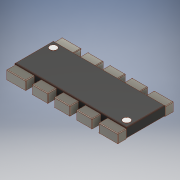
# Autodesk Inventor part: ResistorArray-3264
Saved by Autodesk Inventor 2018 (Build 220112000, 112)
## iProperties
Created: 2018-09-29
Part Number: ResistorArray-3264
Material: Copper
Document SubType Name: Modeling
Designer: Bradley
Density: 8.94 g/cm^3
Appearance: Copper - Satin
Author: Bradley
Autodesk Inventor part; units mm, degrees
ref_plane "YZ Plane" through (0, 0, 0) normal (1, 0, 0) x (0, 1, 0)
ref_plane "XZ Plane" through (0, 0, 0) normal (0, 1, 0) x (-1, 0, 0)
ref_plane "XY Plane" through (0, 0, 0) normal (0, 0, 1) x (1, 0, 0)
sketch "Sketch1" plane through (0, 0, 0) normal (0, 0, 1) x (1, 0, 0)
  line L0 (-3.2, -1.1) -> (3.2, -1.1)
  line L1 (3.2, -1.1) -> (3.2, 1.1)
  line L2 (3.2, 1.1) -> (-3.2, 1.1)
  line L3 (-3.2, 1.1) -> (-3.2, -1.1)
  line L4 (-3.2, -1.1) -> (3.2, 1.1) construction
  line L5 (3.2, -1.1) -> (-3.2, 1.1) construction
  point P0 (0, 0)
  dimension "d0" = 6.4
  dimension "d1" = 2.2
  constraints: 12 end point, 2 midpoint, 2 parallel, 1 horizontal, 1 perpendicular
  measures "d0" distance of L2.end L1.end
  measures "d1" distance of L2.end L0.start
extrude "Extrusion1" add sketch "Sketch1" along normal mid plane 0.55
sketch "Sketch2" plane through (0, 0, 0) normal (0, 0, 1) x (1, 0, 0)
  line L0 (-3.2, -1.1) -> (3.2, -1.1) projected
  line L1 (3.2, -1.1) -> (3.2, 1.1) projected
  line L2 (3.2, 1.1) -> (-3.2, 1.1) projected
  line L3 (-3.2, 1.1) -> (-3.2, -1.1) projected
  line L4 (3.2, 1.1) -> (-3.2, 1.1) projected
  line L5 (-3.19, 1.1) -> (-2.09, 1.1)
  line L6 (-2.09, 1.1) -> (-2.09, 1.6)
  line L7 (-2.09, 1.6) -> (-3.19, 1.6)
  line L8 (-3.19, 1.6) -> (-3.19, 1.1)
  line L9 (-3.19, -1.1) -> (-2.09, -1.1)
  line L10 (-2.09, -1.1) -> (-2.09, -1.6)
  line L11 (-2.09, -1.6) -> (-3.19, -1.6)
  line L12 (-3.19, -1.6) -> (-3.19, -1.1)
  line L13 (3.19, -1.1) -> (2.09, -1.1)
  line L14 (2.09, -1.1) -> (2.09, -1.6)
  line L15 (2.09, -1.6) -> (3.19, -1.6)
  line L16 (3.19, -1.6) -> (3.19, -1.1)
  line L17 (3.19, 1.1) -> (2.09, 1.1)
  line L18 (2.09, 1.1) -> (2.09, 1.6)
  line L19 (2.09, 1.6) -> (3.19, 1.6)
  line L20 (3.19, 1.6) -> (3.19, 1.1)
  line L21 (-1.72, 1.1) -> (-0.82, 1.1)
  line L22 (-0.82, 1.1) -> (-0.82, 1.6)
  line L23 (-0.82, 1.6) -> (-1.72, 1.6)
  line L24 (-1.72, 1.6) -> (-1.72, 1.1)
  line L25 (-3.2, -1.1) -> (3.2, -1.1) projected
  line L26 (-1.72, -1.1) -> (-0.82, -1.1)
  line L27 (-0.82, -1.1) -> (-0.82, -1.6)
  line L28 (-0.82, -1.6) -> (-1.72, -1.6)
  line L29 (-1.72, -1.6) -> (-1.72, -1.1)
  line L30 (-0.45, -1.1) -> (0.45, -1.1)
  line L31 (0.45, -1.1) -> (0.45, -1.6)
  line L32 (0.45, -1.6) -> (-0.45, -1.6)
  line L33 (-0.45, -1.6) -> (-0.45, -1.1)
  line L34 (0.45, 1.6) -> (-0.45, 1.6)
  line L35 (-0.45, 1.6) -> (-0.45, 1.1)
  line L36 (0.45, 1.1) -> (0.45, 1.6)
  line L37 (-0.45, 1.1) -> (0.45, 1.1)
  line L38 (0.82, -1.1) -> (1.72, -1.1)
  line L39 (1.72, -1.1) -> (1.72, -1.6)
  line L40 (1.72, -1.6) -> (0.82, -1.6)
  line L41 (0.82, -1.6) -> (0.82, -1.1)
  line L42 (1.72, 1.6) -> (0.82, 1.6)
  line L43 (0.82, 1.6) -> (0.82, 1.1)
  line L44 (1.72, 1.1) -> (1.72, 1.6)
  line L45 (0.82, 1.1) -> (1.72, 1.1)
  point P0 (0, 0)
  point P1 (0, 1.1)
  dimension "d4" = 1.1
  dimension "d5" = 0.9
  dimension "d6" = 3.2
  dimension "d9" = 1.27
  dimension "d18" = 0.01
  dimension "d19" = 0.01
  constraints: 80 end point, 14 point on line, 12 parallel, 7 horizontal, 6 perpendicular, 5 collinear, 4 equal length, 2 midpoint, 31 other
  measures "d4" distance of L6.end L7.end
  measures "d5" distance of L22.end L23.end
  measures "d6" distance between parallel lines of L11 L7
  measures "d9" distance of L26.end L30.end
  measures "d18" distance between parallel lines of L1 L20
  measures "d19" distance between parallel lines of L3 L8
extrude "Extrusion2" add sketch "Sketch2" along normal blind 0.2 and the other way blind 0.325 contours L0 L10 L11 L12 | L8 L7 L6 L2 | L0 L27 L28 L29 | L24 L23 L22 L2 | L0 L31 L32 L33 | L35 L34 L36 L2 | L0 L39 L40 L41 | L43 L42 L44 L2 | L0 L16 L15 L14 | L18 L19 L20 L2
sketch "Sketch3" plane through (0, 0, 0.275) normal (0, 0, 1) x (1, 0, 0)
  circle A0 centre (-2.85, 0.75) radius 0.2
  circle A1 centre (2.85, -0.75) radius 0.2
  line L0 (-3.2, -1.1) -> (3.2, -1.1) projected
  line L1 (3.2, -1.1) -> (3.2, 1.1) projected
  line L2 (3.2, 1.1) -> (-3.2, 1.1) projected
  line L3 (-3.2, 1.1) -> (-3.2, -1.1) projected
  circle A2 centre (-2.85, 0.75) radius 0.35 construction
  circle A3 centre (2.85, -0.75) radius 0.35 construction
  point P0 (0, 0)
  dimension "d20" = 0.4
  dimension "d21" = 0.7
  constraints: 4 centre point, 4 tangent, 2 coincident, 2 equal radius
  measures "d20" diameter of A0
  measures "d21" diameter of A2
extrude "Extrusion3" add sketch "Sketch3" along normal blind 0.01 contours A0 | A1
fillet "Fillet1" radius 0.03 110 edges at (-2.09, -1.35, -0.325) (-2.64, -1.6, -0.325) (-3.19, -1.35, -0.325) (-2.64, -1.1, -0.325) (-2.09, -1.6, -0.0625) (-2.64, -1.6, 0.2) (-3.19, -1.6, -0.0625) (-3.19, -1.35, 0.2) (-3.19, -1.1, -0.3) (-2.09, -1.1, -0.3) (-2.09, -1.35, 0.2) (-2.64, 1.1, -0.325) (-3.19, 1.35, -0.325) (-2.64, 1.6, -0.325) (-2.09, 1.35, -0.325) (-3.19, 1.35, 0.2) (-3.19, 1.6, -0.0625) (-3.19, 1.1, -0.3) (-2.64, 1.6, 0.2) (-2.09, 1.6, -0.0625) (-2.09, 1.35, 0.2) (-2.09, 1.1, -0.3) (1.27, -1.1, -0.325) (1.72, -1.35, -0.325) (1.27, -1.6, -0.325) (0.82, -1.35, -0.325) (1.72, -1.35, 0.2) (1.72, -1.6, -0.0625) (1.72, -1.1, -0.3) (1.27, -1.6, 0.2) (0.82, -1.6, -0.0625) (0.82, -1.35, 0.2) (0.82, -1.1, -0.3) (-1.27, 1.1, -0.325) (-1.72, 1.35, -0.325) (-1.27, 1.6, -0.325) (-0.82, 1.35, -0.325) (-1.72, 1.35, 0.2) (-1.72, 1.6, -0.0625) (-1.72, 1.1, -0.3) (-1.27, 1.6, 0.2) (-0.82, 1.6, -0.0625) (-0.82, 1.35, 0.2) (-0.82, 1.1, -0.3) (-0.82, -1.1, -0.3) (-1.27, -1.1, -0.325) (-1.72, -1.1, -0.3) (-1.72, -1.35, -0.325) (-0.82, -1.35, -0.325) (-1.27, -1.6, -0.325) (-0.82, -1.35, 0.2) (-0.82, -1.6, -0.0625) (-1.27, -1.6, 0.2) (-1.72, -1.6, -0.0625) (-1.72, -1.35, 0.2) (0, 1.1, -0.325) (-0.45, 1.35, -0.325) (0, 1.6, -0.325) (0.45, 1.35, -0.325) (-0.45, 1.1, -0.3) (-0.45, 1.35, 0.2) (-0.45, 1.6, -0.0625) (0, 1.6, 0.2) (0.45, 1.6, -0.0625) (0.45, 1.35, 0.2) (0.45, 1.1, -0.3) (0, -1.1, -0.325) (0.45, -1.35, -0.325) (0, -1.6, -0.325) (-0.45, -1.35, -0.325) (0.45, -1.35, 0.2) (0.45, -1.6, -0.0625) (0.45, -1.1, -0.3) (0, -1.6, 0.2) (-0.45, -1.6, -0.0625) (-0.45, -1.35, 0.2) (-0.45, -1.1, -0.3) (1.27, 1.1, -0.325) (0.82, 1.35, -0.325) (1.27, 1.6, -0.325) (1.72, 1.35, -0.325) (0.82, 1.35, 0.2) (0.82, 1.6, -0.0625) (0.82, 1.1, -0.3) (1.27, 1.6, 0.2) (1.72, 1.6, -0.0625) (1.72, 1.35, 0.2) (1.72, 1.1, -0.3) (2.09, 1.1, -0.3) (2.64, 1.1, -0.325) (3.19, 1.1, -0.3) (3.19, 1.35, -0.325) (2.09, 1.35, -0.325) (2.64, 1.6, -0.325) (2.09, 1.35, 0.2) (2.09, 1.6, -0.0625) (2.64, 1.6, 0.2) (3.19, 1.6, -0.0625) (3.19, 1.35, 0.2) (3.19, -1.1, -0.3) (2.64, -1.1, -0.325) (2.09, -1.1, -0.3) (2.09, -1.35, -0.325) (3.19, -1.35, -0.325) (2.64, -1.6, -0.325) (3.19, -1.35, 0.2) (3.19, -1.6, -0.0625) (2.64, -1.6, 0.2) (2.09, -1.6, -0.0625) (2.09, -1.35, 0.2)
fillet "Fillet2" radius 0.03 18 edges at (3.195, -1.1, -0.275) (1.905, -1.1, -0.275) (0.635, -1.1, -0.275) (-0.635, -1.1, -0.275) (-1.905, -1.1, -0.275) (-3.195, -1.1, -0.275) (-3.2, 0, -0.275) (-3.195, 1.1, -0.275) (-1.905, 1.1, -0.275) (-0.635, 1.1, -0.275) (0.635, 1.1, -0.275) (1.905, 1.1, -0.275) (3.195, 1.1, -0.275) (3.2, 0, -0.275) (-3.2, 0, 0.275) (0, 1.1, 0.275) (3.2, 0, 0.275) (0, -1.1, 0.275)
equation "\"d19\" = d18"
body "Solid1"
